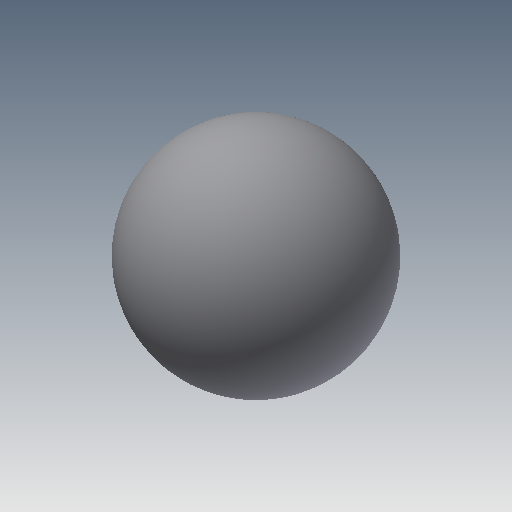
# Autodesk Inventor part: SAR3_ba
Saved by Autodesk Inventor 2020 (Build 240168000, 168)
## iProperties
Created: 2019-11-17
Part Number: SAR3_ba
Material: Generic
Catalog Web Link: www.cadenas.de
Description: SAR3_ball-Slide Rails - Aluminum Alloy - Three - Step Slide Rails
Vendor: MISUMI
Document SubType Name: Modeling
Designer: psadmin
Manufacturer: MISUMI
Mass: 0.0287309 g
Surface Area: 0.453646 cm^2
Volume: 0.0287309 cm^3
Density: 1 g/cm^3
Appearance: PSOLRGB-192-192-192
Category: PARTsolutions
Company: MISUMI
PSOL_IDENT_0: {$CADENAS_DATA\23d-libs\misumi\metric\07_slide_rails\sar3_series\sar3_ball.prj},154 {VTYP=3D},{NB=SA
PSOL_IDENT_1: R3_ba},{LINA=SAR3},{NN=SAR3_ball},{DATE=17.04.2019 06:32:03},{GEOMDATE=16.04.2019 08:26:20},{VERSION=
PSOL_IDENT_2: },{LINEID=10},{WBVAR=},{WBNUMERIC=}  {NB=SAR3_ba},{LINA=SAR3},{KT=DUMMY},{PN=SAR3},{TYPE=SAR3}
NN: SAR3_ball
NT: Slide Rails - Aluminum Alloy - Three - Step Slide Rails
NB: SAR3_ba
NBSYN: $PN._ba
LINA: SAR3
PN: SAR3
TYPE: SAR3
SUPPLIER: MISUMI
ARTICLENO: SAR3_ba
BOMINFO: SAR3
CREATOR: CADENAS GmbH
Title: SAR3
Author: Cadenas PARTsolutions
Comments: Slide Rails - Aluminum Alloy - Three - Step Slide Rails
Autodesk Inventor part; units mm, degrees
sketch "Sketch_2" plane through (0, 0, 0) normal (1, 0, 0) x (0, 1, 0)
  line L0 (0, -1.9) -> (0, 1.9)
  arc A0 (0, -1.9) -> (0, 1.9) centre (0, 0) ccw
  line L1 (0, -1.9) -> (0, 1.9)
  constraints: 4 end point, 2 point on circle, 1 centre point
revolve "Revolution1" add sketch "Sketch_2" angle 360 about axis through (0, 0, -1.9) along (0, 0, -1)
ref_plane "to_rail_XY" through (0, 0, 0) normal (1, 0, 0) x (0, 0, -1)
ref_plane "to_rail_YZ" through (0, 0, 0) normal (0, 0, -1) x (0, 1, 0)
ref_plane "to_rail_ZX" through (0, 0, 0) normal (0, 1, 0) x (1, 0, 0)
body "Solid1"
